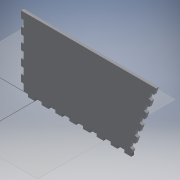
# Autodesk Inventor part: боковушка
Saved by Autodesk Inventor 2019 (Build 230136000, 136)
## iProperties
Created: 2022-06-29
Part Number: боковушка
Material: Типовые
Document SubType Name: Modeling
Designer: korsh
Density: 1 g/cm^3
Appearance: По умолчанию
Author: korsh
Autodesk Inventor part; units mm, degrees
ref_plane "YZ Plane" through (0, 0, 0) normal (1, 0, 0) x (0, 1, 0)
ref_plane "XZ Plane" through (0, 0, 0) normal (0, 1, 0) x (-1, 0, 0)
ref_plane "XY Plane" through (0, 0, 0) normal (0, 0, 1) x (1, 0, 0)
sketch "Эскиз1" plane through (0, 0, 0) normal (0, 0, 1) x (1, 0, 0)
  line L0 (130, 0) -> (130, 4) projected
  line L1 (140, 4) -> (130, 4) projected
  line L2 (140, 0) -> (140, 4) projected
  line L3 (140, 0) -> (130, 0) projected
  line L4 (120, 0) -> (120, 4) projected
  line L5 (120, 4) -> (110, 4) projected
  line L6 (110, 4) -> (110, 0) projected
  line L7 (120, 0) -> (110, 0) projected
  line L8 (90, 4) -> (90, 0) projected
  line L9 (100, 0) -> (90, 0) projected
  line L10 (100, 0) -> (100, 4) projected
  line L11 (100, 4) -> (90, 4) projected
  line L12 (80, 0) -> (80, 4) projected
  line L13 (80, 4) -> (70, 4) projected
  line L14 (70, 4) -> (70, 0) projected
  line L15 (80, 0) -> (70, 0) projected
  line L16 (50, 4) -> (50, 0) projected
  line L17 (60, 0) -> (50, 0) projected
  line L18 (60, 0) -> (60, 4) projected
  line L19 (60, 4) -> (50, 4) projected
  line L20 (40, 0) -> (40, 4) projected
  line L21 (40, 4) -> (30, 4) projected
  line L22 (30, 4) -> (30, 0) projected
  line L23 (40, 0) -> (30, 0) projected
  line L24 (10, 4) -> (10, 0) projected
  line L25 (20, 0) -> (10, 0) projected
  line L26 (20, 0) -> (20, 4) projected
  line L27 (20, 4) -> (10, 4) projected
  line L28 (0, 0) -> (0, 4) projected
  line L29 (0, 4) -> (-10, 4) projected
  line L30 (-10, 4) -> (-10, 0) projected
  line L31 (0, 0) -> (-10, 0) projected
  line L32 (-20, 4) -> (-10, 4) projected
  line L33 (-20, 4) -> (140, 4)
  line L34 (-20, 4) -> (-20, 104)
  line L35 (140, 4) -> (176.397, 104)
  line L36 (140, 4) -> (246.4178, 4) construction
  line L37 (176.397, 104) -> (-20, 104)
  line L38 (-20, 94) -> (-16, 94)
  line L39 (-16, 94) -> (-16, 84)
  line L40 (-16, 84) -> (-20, 84)
  line L41 (-20, 84) -> (-20, 94)
  line L42 (-16, 74) -> (-16, 64)
  line L43 (-20, 64) -> (-20, 74)
  line L44 (-20, 74) -> (-16, 74)
  line L45 (-16, 64) -> (-20, 64)
  line L46 (-16, 54) -> (-16, 44)
  line L47 (-20, 44) -> (-20, 54)
  line L48 (-20, 54) -> (-16, 54)
  line L49 (-16, 44) -> (-20, 44)
  line L50 (-16, 34) -> (-16, 24)
  line L51 (-20, 24) -> (-20, 34)
  line L52 (-20, 34) -> (-16, 34)
  line L53 (-16, 24) -> (-20, 24)
  line L54 (-16, 14) -> (-16, 4)
  line L55 (-20, 4) -> (-20, 14)
  line L56 (-20, 14) -> (-16, 14)
  line L57 (-16, 4) -> (-20, 4)
  line L58 (172.7573, 94) -> (169.3371, 84.6031)
  line L59 (169.3371, 84.6031) -> (165.5783, 85.9712)
  line L60 (165.5783, 85.9712) -> (168.9986, 95.3681)
  line L61 (168.9986, 95.3681) -> (172.7573, 94)
  line L62 (158.7379, 67.1773) -> (162.1581, 76.5742)
  line L63 (165.9169, 75.2061) -> (162.4967, 65.8092)
  line L64 (162.1581, 76.5742) -> (165.9169, 75.2061)
  line L65 (162.4967, 65.8092) -> (158.7379, 67.1773)
  line L66 (151.8975, 48.3834) -> (155.3177, 57.7804)
  line L67 (159.0765, 56.4123) -> (155.6563, 47.0154)
  line L68 (155.3177, 57.7804) -> (159.0765, 56.4123)
  line L69 (155.6563, 47.0154) -> (151.8975, 48.3834)
  line L70 (145.0571, 29.5896) -> (148.4773, 38.9865)
  line L71 (152.2361, 37.6184) -> (148.8159, 28.2215)
  line L72 (148.4773, 38.9865) -> (152.2361, 37.6184)
  line L73 (148.8159, 28.2215) -> (145.0571, 29.5896)
  line L74 (138.2167, 10.7957) -> (141.6369, 20.1927)
  line L75 (145.3957, 18.8246) -> (141.9755, 9.4277)
  line L76 (141.6369, 20.1927) -> (145.3957, 18.8246)
  line L77 (141.9755, 9.4277) -> (138.2167, 10.7957)
  dimension "d0" = 100
  dimension "d1" = 70
  dimension "d2" = 4
  dimension "d3" = 10
  dimension "d4" = 10
  dimension "d7" = 20
  dimension "d12" = 10
  dimension "d13" = 4
  dimension "d14" = 10
  dimension "d17" = 20
  constraints: 90 end point, 4 horizontal, 4 perpendicular, 3 point on line, 2 parallel, 1 equal length, 1 vertical, 65 other
  measures "d0" distance of L32.start L34.end
  measures "d1" angle of L36 L35
  measures "d2" distance of L39.end L40.end
  measures "d3" distance of L38.end L39.end
  measures "d4" distance from line of L38 L34.end
  measures "d7" distance of L39.end L42.end
  measures "d12" distance of L58.start L58.end
  measures "d13" distance of L58.end L59.end
  measures "d14" distance of L59.end L60.end
  measures "d17" distance of L60.end L62.end
extrude "Выдавливание1" add sketch "Эскиз1" along normal blind 4 contours L0 L1 L2 L3 | L33 L5 L11 L13 L19 L21 L27 L29 L32 L54 L56 L34 L53 L50 L52 L49 L46 L48 L45 L42 L44 L40 L39 L38 L37 L35 L61 L60 L59 L64 L62 L65 L68 L66 L69 L72 L70 L73 L76 L74 L77 L1 | L4 L7 L6 L5 | L10 L9 L8 L11 | L12 L15 L14 L13 | L18 L17 L16 L19 | L20 L23 L22 L21 | L26 L25 L24 L27 | L28 L31 L30 L29
